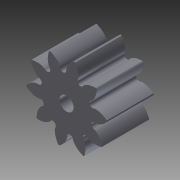
# Autodesk Inventor part: 276-2181-004 Rev1
Saved by Autodesk Inventor 2013 (Build 170138000, 138)
## iProperties
Category: Motors
Company: Autodesk Inc.
Created: 2012-01-24
Part Number: 276-2181-004 Rev1
Material: Steel
Document SubType Name: Modeling
Designer: Autodesk Inc.
Density: 7.85 g/cm^3
Catalog Web Link: http://www.vexrobotics.com/276-2181.html
Vendor: VEX
Mass: 0.321197 g
Surface Area: 1.10628 cm^2
Volume: 0.0409168 cm^3
Author: Autodesk Inc.
Autodesk Inventor part; units mm, degrees
(part 1 of 2)
ref_plane "YZ Plane" through (0, 0, 0) normal (1, 0, 0) x (0, 1, 0)
ref_plane "XZ Plane" through (0, 0, 0) normal (0, 1, 0) x (-1, 0, 0)
ref_plane "XY Plane" through (0, 0, 0) normal (0, 0, 1) x (1, 0, 0)
sketch "Sketch1" plane through (0, 0, 0) normal (0, 0, 1) x (1, 0, 0)
  spline S0 degree 3 poles (1.9335, 1.7383) (1.9334, 1.7374) (1.9328, 1.7292) (1.9315, 1.7139) (1.9295, 1.6925) (1.9272, 1.6714) (1.9247, 1.6506) (1.9219, 1.6301) (1.919, 1.6099) (1.9159, 1.59) (1.9125, 1.5704) (1.909, 1.5512) (1.9053, 1.5323) (1.9014, 1.5137) (1.8974, 1.4954) (1.8932, 1.4775) (1.8888, 1.4598) (1.8843, 1.4426) (1.8797, 1.4256) (1.8749, 1.4089) (1.87, 1.3926) (1.865, 1.3767) (1.8599, 1.361) (1.8547, 1.3457) (1.8494, 1.3307) (1.844, 1.316) (1.8385, 1.3017) (1.833, 1.2877) (1.8274, 1.274) (1.8217, 1.2607) (1.816, 1.2477) (1.8103, 1.235) (1.8045, 1.2226) (1.7987, 1.2106) (1.7928, 1.1989) (1.787, 1.1875) (1.7811, 1.1764) (1.7753, 1.1657) (1.7694, 1.1553) (1.7636, 1.1452) (1.7577, 1.1354) (1.7519, 1.1259) (1.7462, 1.1167) (1.7405, 1.1078) (1.7348, 1.0993) (1.7292, 1.091) (1.7236, 1.083) (1.7181, 1.0754) (1.7127, 1.068) (1.7074, 1.0609) (1.7021, 1.0541) (1.697, 1.0476) (1.6919, 1.0414) (1.687, 1.0355) (1.6821, 1.0298) (1.6774, 1.0244) (1.6728, 1.0193) (1.6683, 1.0144) (1.664, 1.0098) (1.6598, 1.0054) (1.6557, 1.0013) (1.6518, 0.9975) (1.648, 0.9939) (1.6444, 0.9905) (1.641, 0.9874) (1.6378, 0.9845) (1.6347, 0.9818) (1.6318, 0.9793) (1.6291, 0.9771) (1.6266, 0.975) (1.6242, 0.9732) (1.6221, 0.9716) (1.6202, 0.9702) (1.6185, 0.9689) (1.617, 0.9678) (1.6107, 0.9635) (1.5995, 0.9583) (1.585, 0.9495) (1.5719, 0.9412) (1.5594, 0.9325) (1.5474, 0.9234) (1.5359, 0.9137) (1.5249, 0.9036) (1.5144, 0.8928) (1.5044, 0.8812) (1.495, 0.8687) (1.4861, 0.8551) (1.478, 0.8401) (1.4709, 0.8236) (1.4651, 0.8052) (1.461, 0.7849) (1.4595, 0.7627) (1.4612, 0.739) (1.4666, 0.716) (1.4733, 0.6979) (1.4797, 0.6848) (1.4855, 0.6714) (1.495, 0.6545) (1.5091, 0.6356) (1.5261, 0.619) (1.544, 0.6057) (1.562, 0.5956) (1.5798, 0.5882) (1.597, 0.583) (1.6137, 0.5795) (1.6298, 0.5774) (1.6454, 0.5765) (1.6607, 0.5766) (1.6757, 0.5776) (1.6906, 0.5794) (1.7054, 0.5819) (1.7201, 0.5852) (1.7349, 0.5891) (1.7496, 0.5937) (1.7657, 0.5991) (1.7769, 0.6043) (1.7844, 0.6062) (1.7861, 0.6067) (1.7882, 0.6072) (1.7905, 0.6077) (1.7931, 0.6083) (1.796, 0.6089) (1.7992, 0.6095) (1.8027, 0.6101) (1.8064, 0.6107) (1.8105, 0.6113) (1.8148, 0.6119) (1.8194, 0.6125) (1.8243, 0.613) (1.8295, 0.6136) (1.8349, 0.614) (1.8407, 0.6145) (1.8467, 0.6149) (1.853, 0.6152) (1.8596, 0.6155) (1.8665, 0.6157) (1.8737, 0.6158) (1.8812, 0.6158) (1.8889, 0.6157) (1.8969, 0.6156) (1.9052, 0.6153) (1.9138, 0.6149) (1.9227, 0.6144) (1.9318, 0.6137) (1.9412, 0.613) (1.9508, 0.612) (1.9608, 0.611) (1.971, 0.6098) (1.9814, 0.6084) (1.9922, 0.6068) (2.0031, 0.6051) (2.0144, 0.6032) (2.0259, 0.6011) (2.0376, 0.5988) (2.0496, 0.5963) (2.0618, 0.5936) (2.0743, 0.5907) (2.087, 0.5876) (2.0999, 0.5842) (2.1131, 0.5807) (2.1265, 0.5768) (2.1401, 0.5728) (2.1539, 0.5684) (2.168, 0.5639) (2.1823, 0.559) (2.1967, 0.5539) (2.2114, 0.5485) (2.2262, 0.5429) (2.2413, 0.5369) (2.2565, 0.5307) (2.2719, 0.5242) (2.2875, 0.5174) (2.3033, 0.5102) (2.3192, 0.5028) (2.3353, 0.495) (2.3516, 0.4869) (2.368, 0.4785) (2.3845, 0.4698) (2.4012, 0.4607) (2.418, 0.4513) (2.435, 0.4415) (2.4521, 0.4314) (2.4692, 0.4209) (2.4865, 0.4101) (2.5039, 0.3989) (2.5214, 0.3873) (2.539, 0.3754) (2.5574, 0.3626) (2.5699, 0.3536) (2.5765, 0.3488) knots 0.016719 0.016719 0.016719 0.016719 0.017808 0.026543 0.035166 0.043676 0.052073 0.060357 0.068528 0.076587 0.084533 0.092367 0.100087 0.107695 0.115191 0.122573 0.129843 0.137 0.144045 0.150977 0.157796 0.164502 0.171095 0.177576 0.183945 0.1902 0.196343 0.202373 0.20829 0.214095 0.219787 0.225366 0.230832 0.236186 0.241427 0.246556 0.251571 0.256474 0.261264 0.265942 0.270507 0.274959 0.279298 0.283525 0.287639 0.29164 0.295528 0.299304 0.302967 0.306518 0.309956 0.31328 0.316493 0.319592 0.322579 0.325453 0.328215 0.330863 0.333399 0.335823 0.338133 0.340331 0.342416 0.344389 0.346248 0.347996 0.34963 0.351151 0.35256 0.353856 0.35504 0.356111 0.357069 0.357914 0.358647 0.359267 0.367127 0.373439 0.379636 0.385738 0.391769 0.397757 0.403738 0.409752 0.415852 0.422098 0.428563 0.435333 0.442503 0.450171 0.458425 0.467319 0.476841 0.486882 0.495598 0.5 0.504402 0.513118 0.523159 0.532681 0.541575 0.549829 0.557497 0.564667 0.571437 0.577902 0.584148 0.590248 0.596262 0.602243 0.608231 0.614262 0.620364 0.626561 0.632873 0.640733 0.641353 0.642086 0.642931 0.643889 0.64496 0.646144 0.64744 0.648849 0.65037 0.652004 0.653752 0.655611 0.657584 0.659669 0.661867 0.664177 0.666601 0.669137 0.671785 0.674547 0.677421 0.680408 0.683507 0.68672 0.690044 0.693482 0.697033 0.700696 0.704472 0.70836 0.712361 0.716475 0.720702 0.725041 0.729493 0.734058 0.738736 0.743526 0.748429 0.753444 0.758573 0.763814 0.769168 0.774634 0.780213 0.785905 0.79171 0.797627 0.803657 0.8098 0.816055 0.822424 0.828905 0.835498 0.842204 0.849023 0.855955 0.863 0.870157 0.877427 0.884809 0.892305 0.899913 0.907633 0.915467 0.923413 0.931472 0.939643 0.947927 0.956324 0.964834 0.973457 0.983281 0.983281 0.983281 0.983281
  arc A0 (1.9335, 1.7383) -> (1.8794, 1.7966) centre (0, 0) ccw
  spline S1 degree 3 poles (0.5425, 2.5428) (0.543, 2.542) (0.5472, 2.535) (0.5552, 2.5219) (0.5661, 2.5034) (0.5767, 2.4849) (0.5869, 2.4666) (0.5968, 2.4484) (0.6063, 2.4304) (0.6154, 2.4125) (0.6242, 2.3947) (0.6327, 2.377) (0.6408, 2.3596) (0.6486, 2.3422) (0.656, 2.3251) (0.6632, 2.3081) (0.67, 2.2913) (0.6765, 2.2746) (0.6828, 2.2582) (0.6887, 2.2419) (0.6943, 2.2259) (0.6997, 2.21) (0.7047, 2.1943) (0.7095, 2.1789) (0.714, 2.1636) (0.7183, 2.1486) (0.7223, 2.1338) (0.726, 2.1192) (0.7295, 2.1048) (0.7328, 2.0907) (0.7358, 2.0768) (0.7386, 2.0632) (0.7412, 2.0498) (0.7436, 2.0366) (0.7457, 2.0237) (0.7477, 2.0111) (0.7495, 1.9987) (0.751, 1.9865) (0.7524, 1.9747) (0.7536, 1.963) (0.7547, 1.9517) (0.7556, 1.9406) (0.7563, 1.9298) (0.7569, 1.9193) (0.7574, 1.909) (0.7577, 1.899) (0.7579, 1.8893) (0.7579, 1.8799) (0.7579, 1.8707) (0.7577, 1.8619) (0.7575, 1.8533) (0.7571, 1.845) (0.7567, 1.837) (0.7561, 1.8293) (0.7556, 1.8218) (0.7549, 1.8147) (0.7542, 1.8078) (0.7534, 1.8013) (0.7526, 1.795) (0.7518, 1.789) (0.7509, 1.7833) (0.75, 1.7779) (0.7491, 1.7728) (0.7482, 1.7679) (0.7472, 1.7634) (0.7463, 1.7591) (0.7454, 1.7551) (0.7445, 1.7514) (0.7436, 1.748) (0.7428, 1.7449) (0.742, 1.7421) (0.7412, 1.7395) (0.7405, 1.7372) (0.7399, 1.7352) (0.7393, 1.7335) (0.7368, 1.7262) (0.7307, 1.7154) (0.7242, 1.6998) (0.7184, 1.6854) (0.7134, 1.671) (0.7091, 1.6565) (0.7055, 1.642) (0.7026, 1.6273) (0.7004, 1.6124) (0.6992, 1.5972) (0.6989, 1.5815) (0.6997, 1.5653) (0.7019, 1.5484) (0.7059, 1.5309) (0.7119, 1.5126) (0.7206, 1.4938) (0.7325, 1.4749) (0.7478, 1.4567) (0.7656, 1.4413) (0.7817, 1.4306) (0.7946, 1.4237) (0.8072, 1.4164) (0.8247, 1.4083) (0.8473, 1.4012) (0.8708, 1.3977) (0.8931, 1.3976) (0.9136, 1.4) (0.9323, 1.4045) (0.9494, 1.4103) (0.9649, 1.4173) (0.9791, 1.4251) (0.9923, 1.4335) (1.0046, 1.4426) (1.0162, 1.4523) (1.0272, 1.4625) (1.0376, 1.4732) (1.0476, 1.4845) (1.0573, 1.4963) (1.0665, 1.5087) (1.0764, 1.5225) (1.0824, 1.5333) (1.0872, 1.5393) (1.0884, 1.5407) (1.0898, 1.5423) (1.0914, 1.5441) (1.0931, 1.5461) (1.0951, 1.5483) (1.0974, 1.5506) (1.0998, 1.5531) (1.1025, 1.5558) (1.1054, 1.5587) (1.1085, 1.5617) (1.1119, 1.5649) (1.1155, 1.5682) (1.1194, 1.5717) (1.1236, 1.5753) (1.128, 1.5791) (1.1326, 1.5829) (1.1375, 1.5869) (1.1427, 1.591) (1.1482, 1.5952) (1.1539, 1.5995) (1.1599, 1.6039) (1.1662, 1.6084) (1.1728, 1.613) (1.1797, 1.6176) (1.1869, 1.6224) (1.1943, 1.6271) (1.2021, 1.632) (1.2101, 1.6369) (1.2185, 1.6418) (1.2272, 1.6468) (1.2361, 1.6518) (1.2454, 1.6568) (1.255, 1.6619) (1.2649, 1.6669) (1.2751, 1.672) (1.2856, 1.6771) (1.2965, 1.6821) (1.3076, 1.6872) (1.3191, 1.6922) (1.3309, 1.6971) (1.343, 1.7021) (1.3555, 1.707) (1.3682, 1.7118) (1.3813, 1.7166) (1.3947, 1.7213) (1.4085, 1.7259) (1.4225, 1.7305) (1.4369, 1.735) (1.4516, 1.7393) (1.4666, 1.7436) (1.482, 1.7478) (1.4976, 1.7518) (1.5136, 1.7557) (1.5299, 1.7595) (1.5466, 1.7631) (1.5635, 1.7666) (1.5808, 1.77) (1.5984, 1.7731) (1.6163, 1.7762) (1.6345, 1.779) (1.653, 1.7816) (1.6718, 1.7841) (1.691, 1.7864) (1.7104, 1.7884) (1.7302, 1.7903) (1.7502, 1.7919) (1.7706, 1.7933) (1.7912, 1.7945) (1.8122, 1.7954) (1.8334, 1.7961) (1.8559, 1.7965) (1.8712, 1.7966) (1.8794, 1.7966) knots 0.016719 0.016719 0.016719 0.016719 0.017808 0.026543 0.035166 0.043676 0.052073 0.060357 0.068528 0.076587 0.084533 0.092367 0.100087 0.107695 0.115191 0.122573 0.129843 0.137 0.144045 0.150977 0.157796 0.164502 0.171095 0.177576 0.183945 0.1902 0.196343 0.202373 0.20829 0.214095 0.219787 0.225366 0.230832 0.236186 0.241427 0.246556 0.251571 0.256474 0.261264 0.265942 0.270507 0.274959 0.279298 0.283525 0.287639 0.29164 0.295528 0.299304 0.302967 0.306518 0.309956 0.31328 0.316493 0.319592 0.322579 0.325453 0.328215 0.330863 0.333399 0.335823 0.338133 0.340331 0.342416 0.344389 0.346248 0.347996 0.34963 0.351151 0.35256 0.353856 0.35504 0.356111 0.357069 0.357914 0.358647 0.359267 0.367127 0.373439 0.379636 0.385738 0.391769 0.397757 0.403738 0.409752 0.415852 0.422098 0.428563 0.435333 0.442503 0.450171 0.458425 0.467319 0.476841 0.486882 0.495598 0.5 0.504402 0.513118 0.523159 0.532681 0.541575 0.549829 0.557497 0.564667 0.571437 0.577902 0.584148 0.590248 0.596262 0.602243 0.608231 0.614262 0.620364 0.626561 0.632873 0.640733 0.641353 0.642086 0.642931 0.643889 0.64496 0.646144 0.64744 0.648849 0.65037 0.652004 0.653752 0.655611 0.657584 0.659669 0.661867 0.664177 0.666601 0.669137 0.671785 0.674547 0.677421 0.680408 0.683507 0.68672 0.690044 0.693482 0.697033 0.700696 0.704472 0.70836 0.712361 0.716475 0.720702 0.725041 0.729493 0.734058 0.738736 0.743526 0.748429 0.753444 0.758573 0.763814 0.769168 0.774634 0.780213 0.785905 0.79171 0.797627 0.803657 0.8098 0.816055 0.822424 0.828905 0.835498 0.842204 0.849023 0.855955 0.863 0.870157 0.877427 0.884809 0.892305 0.899913 0.907633 0.915467 0.923413 0.931472 0.939643 0.947927 0.956324 0.964834 0.973457 0.983281 0.983281 0.983281 0.983281
  arc A1 (0.5425, 2.5428) -> (0.4644, 2.5582) centre (0, 0) ccw
  spline S2 degree 3 poles (-1.0557, 2.376) (-1.0549, 2.3757) (-1.0473, 2.3726) (-1.0332, 2.3666) (-1.0134, 2.358) (-0.994, 2.3493) (-0.975, 2.3405) (-0.9564, 2.3316) (-0.9381, 2.3226) (-0.9201, 2.3134) (-0.9026, 2.3042) (-0.8854, 2.2949) (-0.8685, 2.2856) (-0.852, 2.2761) (-0.8359, 2.2666) (-0.8201, 2.2571) (-0.8047, 2.2475) (-0.7897, 2.2379) (-0.775, 2.2282) (-0.7606, 2.2186) (-0.7466, 2.2089) (-0.733, 2.1992) (-0.7197, 2.1895) (-0.7067, 2.1798) (-0.6941, 2.1701) (-0.6818, 2.1604) (-0.6699, 2.1508) (-0.6583, 2.1412) (-0.647, 2.1317) (-0.6361, 2.1222) (-0.6254, 2.1127) (-0.6152, 2.1033) (-0.6052, 2.094) (-0.5955, 2.0847) (-0.5862, 2.0756) (-0.5772, 2.0665) (-0.5685, 2.0575) (-0.5601, 2.0486) (-0.552, 2.0398) (-0.5441, 2.0311) (-0.5366, 2.0226) (-0.5294, 2.0141) (-0.5224, 2.0058) (-0.5158, 1.9976) (-0.5094, 1.9896) (-0.5033, 1.9817) (-0.4974, 1.9739) (-0.4918, 1.9664) (-0.4865, 1.9589) (-0.4814, 1.9517) (-0.4766, 1.9446) (-0.472, 1.9377) (-0.4676, 1.9309) (-0.4635, 1.9244) (-0.4596, 1.918) (-0.4559, 1.9118) (-0.4525, 1.9059) (-0.4492, 1.9001) (-0.4462, 1.8946) (-0.4433, 1.8892) (-0.4407, 1.8841) (-0.4382, 1.8792) (-0.436, 1.8745) (-0.4339, 1.87) (-0.432, 1.8658) (-0.4302, 1.8618) (-0.4286, 1.8581) (-0.4271, 1.8546) (-0.4258, 1.8513) (-0.4247, 1.8483) (-0.4237, 1.8455) (-0.4228, 1.843) (-0.422, 1.8407) (-0.4213, 1.8387) (-0.4208, 1.837) (-0.4186, 1.8296) (-0.4171, 1.8173) (-0.4133, 1.8008) (-0.4094, 1.7858) (-0.405, 1.7712) (-0.4, 1.757) (-0.3944, 1.7431) (-0.3881, 1.7295) (-0.3811, 1.7162) (-0.3732, 1.7031) (-0.3642, 1.6902) (-0.354, 1.6776) (-0.3423, 1.6653) (-0.3287, 1.6534) (-0.3131, 1.6422) (-0.295, 1.6321) (-0.2744, 1.6238) (-0.2513, 1.6181) (-0.2278, 1.616) (-0.2084, 1.6168) (-0.194, 1.6189) (-0.1795, 1.6203) (-0.1605, 1.6241) (-0.1381, 1.6316) (-0.1171, 1.6426) (-0.099, 1.6556) (-0.0838, 1.6697) (-0.0712, 1.6843) (-0.0609, 1.699) (-0.0524, 1.7138) (-0.0455, 1.7284) (-0.0398, 1.743) (-0.0352, 1.7576) (-0.0315, 1.7722) (-0.0286, 1.7869) (-0.0265, 1.8017) (-0.025, 1.8167) (-0.0241, 1.832) (-0.0239, 1.8475) (-0.0241, 1.8644) (-0.0256, 1.8767) (-0.0252, 1.8844) (-0.0251, 1.8862) (-0.0249, 1.8883) (-0.0247, 1.8907) (-0.0244, 1.8933) (-0.0241, 1.8963) (-0.0236, 1.8995) (-0.0232, 1.903) (-0.0226, 1.9067) (-0.0219, 1.9108) (-0.0211, 1.915) (-0.0203, 1.9196) (-0.0193, 1.9244) (-0.0182, 1.9295) (-0.017, 1.9349) (-0.0156, 1.9405) (-0.0141, 1.9463) (-0.0125, 1.9525) (-0.0107, 1.9588) (-0.0087, 1.9654) (-0.0066, 1.9723) (-0.0043, 1.9794) (-0.0019, 1.9867) (0.0008, 1.9943) (0.0036, 2.0021) (0.0066, 2.0101) (0.0098, 2.0184) (0.0133, 2.0269) (0.0169, 2.0356) (0.0208, 2.0445) (0.0248, 2.0536) (0.0291, 2.0629) (0.0337, 2.0725) (0.0385, 2.0822) (0.0435, 2.0921) (0.0488, 2.1022) (0.0543, 2.1125) (0.0601, 2.1229) (0.0662, 2.1335) (0.0726, 2.1443) (0.0792, 2.1553) (0.0861, 2.1664) (0.0933, 2.1777) (0.1007, 2.1891) (0.1085, 2.2007) (0.1166, 2.2124) (0.125, 2.2242) (0.1337, 2.2361) (0.1427, 2.2482) (0.152, 2.2604) (0.1617, 2.2727) (0.1716, 2.285) (0.1819, 2.2975) (0.1926, 2.3101) (0.2035, 2.3227) (0.2149, 2.3355) (0.2265, 2.3482) (0.2385, 2.3611) (0.2509, 2.374) (0.2636, 2.387) (0.2767, 2.4) (0.2901, 2.413) (0.3039, 2.4261) (0.318, 2.4391) (0.3326, 2.4522) (0.3474, 2.4653) (0.3627, 2.4785) (0.3784, 2.4916) (0.3944, 2.5046) (0.4108, 2.5177) (0.4276, 2.5307) (0.4454, 2.5443) (0.4578, 2.5534) (0.4644, 2.5582) knots 0.016719 0.016719 0.016719 0.016719 0.017808 0.026543 0.035166 0.043676 0.052073 0.060357 0.068528 0.076587 0.084533 0.092367 0.100087 0.107695 0.115191 0.122573 0.129843 0.137 0.144045 0.150977 0.157796 0.164502 0.171095 0.177576 0.183945 0.1902 0.196343 0.202373 0.20829 0.214095 0.219787 0.225366 0.230832 0.236186 0.241427 0.246556 0.251571 0.256474 0.261264 0.265942 0.270507 0.274959 0.279298 0.283525 0.287639 0.29164 0.295528 0.299304 0.302967 0.306518 0.309956 0.31328 0.316493 0.319592 0.322579 0.325453 0.328215 0.330863 0.333399 0.335823 0.338133 0.340331 0.342416 0.344389 0.346248 0.347996 0.34963 0.351151 0.35256 0.353856 0.35504 0.356111 0.357069 0.357914 0.358647 0.359267 0.367127 0.373439 0.379636 0.385738 0.391769 0.397757 0.403738 0.409752 0.415852 0.422098 0.428563 0.435333 0.442503 0.450171 0.458425 0.467319 0.476841 0.486882 0.495598 0.5 0.504402 0.513118 0.523159 0.532681 0.541575 0.549829 0.557497 0.564667 0.571437 0.577902 0.584148 0.590248 0.596262 0.602243 0.608231 0.614262 0.620364 0.626561 0.632873 0.640733 0.641353 0.642086 0.642931 0.643889 0.64496 0.646144 0.64744 0.648849 0.65037 0.652004 0.653752 0.655611 0.657584 0.659669 0.661867 0.664177 0.666601 0.669137 0.671785 0.674547 0.677421 0.680408 0.683507 0.68672 0.690044 0.693482 0.697033 0.700696 0.704472 0.70836 0.712361 0.716475 0.720702 0.725041 0.729493 0.734058 0.738736 0.743526 0.748429 0.753444 0.758573 0.763814 0.769168 0.774634 0.780213 0.785905 0.79171 0.797627 0.803657 0.8098 0.816055 0.822424 0.828905 0.835498 0.842204 0.849023 0.855955 0.863 0.870157 0.877427 0.884809 0.892305 0.899913 0.907633 0.915467 0.923413 0.931472 0.939643 0.947927 0.956324 0.964834 0.973457 0.983281 0.983281 0.983281 0.983281
  arc A2 (-1.0557, 2.376) -> (-1.1279, 2.3426) centre (0, 0) ccw
  spline S3 degree 3 poles (-2.2507, 1.3017) (-2.2498, 1.3019) (-2.2419, 1.3038) (-2.2269, 1.3073) (-2.2059, 1.312) (-2.1851, 1.3164) (-2.1645, 1.3204) (-2.1442, 1.3242) (-2.1241, 1.3276) (-2.1042, 1.3308) (-2.0846, 1.3336) (-2.0652, 1.3362) (-2.0461, 1.3386) (-2.0272, 1.3406) (-2.0085, 1.3424) (-1.9902, 1.344) (-1.9721, 1.3453) (-1.9542, 1.3463) (-1.9367, 1.3472) (-1.9194, 1.3478) (-1.9024, 1.3482) (-1.8856, 1.3483) (-1.8691, 1.3483) (-1.853, 1.3481) (-1.8371, 1.3477) (-1.8215, 1.3471) (-1.8061, 1.3463) (-1.7911, 1.3454) (-1.7764, 1.3443) (-1.762, 1.343) (-1.7478, 1.3416) (-1.734, 1.34) (-1.7204, 1.3383) (-1.7072, 1.3365) (-1.6942, 1.3346) (-1.6816, 1.3326) (-1.6693, 1.3304) (-1.6572, 1.3281) (-1.6455, 1.3258) (-1.6341, 1.3234) (-1.623, 1.3209) (-1.6121, 1.3183) (-1.6016, 1.3156) (-1.5914, 1.313) (-1.5815, 1.3102) (-1.5719, 1.3074) (-1.5627, 1.3046) (-1.5537, 1.3017) (-1.545, 1.2989) (-1.5366, 1.296) (-1.5285, 1.2931) (-1.5207, 1.2902) (-1.5133, 1.2873) (-1.5061, 1.2844) (-1.4992, 1.2816) (-1.4926, 1.2787) (-1.4863, 1.2759) (-1.4803, 1.2732) (-1.4746, 1.2705) (-1.4691, 1.2678) (-1.464, 1.2652) (-1.4591, 1.2627) (-1.4545, 1.2602) (-1.4502, 1.2579) (-1.4462, 1.2556) (-1.4424, 1.2534) (-1.4389, 1.2513) (-1.4356, 1.2493) (-1.4327, 1.2474) (-1.43, 1.2456) (-1.4275, 1.244) (-1.4253, 1.2425) (-1.4233, 1.2411) (-1.4216, 1.2399) (-1.4202, 1.2388) (-1.414, 1.2342) (-1.4056, 1.2251) (-1.3928, 1.214) (-1.3809, 1.2041) (-1.3687, 1.1949) (-1.3563, 1.1863) (-1.3436, 1.1783) (-1.3306, 1.171) (-1.317, 1.1644) (-1.3029, 1.1585) (-1.2881, 1.1534) (-1.2725, 1.1492) (-1.2557, 1.1461) (-1.2378, 1.1444) (-1.2185, 1.1445) (-1.198, 1.147) (-1.1764, 1.1524) (-1.1544, 1.1613) (-1.1341, 1.1735) (-1.119, 1.1855) (-1.1085, 1.1957) (-1.0976, 1.2054) (-1.0845, 1.2195) (-1.0708, 1.2388) (-1.0602, 1.2601) (-1.0532, 1.2812) (-1.0492, 1.3015) (-1.0476, 1.3207) (-1.0479, 1.3387) (-1.0497, 1.3556) (-1.0528, 1.3716) (-1.0567, 1.3867) (-1.0616, 1.4012) (-1.0672, 1.4152) (-1.0735, 1.4288) (-1.0804, 1.4421) (-1.0881, 1.4551) (-1.0963, 1.4679) (-1.1053, 1.4806) (-1.1154, 1.4942) (-1.1238, 1.5032) (-1.128, 1.5097) (-1.1289, 1.5112) (-1.1301, 1.513) (-1.1313, 1.5151) (-1.1326, 1.5174) (-1.1341, 1.52) (-1.1356, 1.5228) (-1.1373, 1.5259) (-1.139, 1.5293) (-1.1408, 1.5329) (-1.1427, 1.5369) (-1.1447, 1.5411) (-1.1468, 1.5456) (-1.1489, 1.5503) (-1.151, 1.5554) (-1.1532, 1.5607) (-1.1554, 1.5663) (-1.1577, 1.5722) (-1.16, 1.5784) (-1.1623, 1.5849) (-1.1646, 1.5917) (-1.167, 1.5988) (-1.1693, 1.6062) (-1.1716, 1.6139) (-1.1739, 1.6218) (-1.1762, 1.6301) (-1.1784, 1.6387) (-1.1806, 1.6476) (-1.1828, 1.6567) (-1.1849, 1.6662) (-1.187, 1.676) (-1.189, 1.6861) (-1.1909, 1.6965) (-1.1927, 1.7071) (-1.1945, 1.7181) (-1.1961, 1.7294) (-1.1977, 1.741) (-1.1992, 1.7528) (-1.2005, 1.765) (-1.2017, 1.7775) (-1.2028, 1.7902) (-1.2037, 1.8033) (-1.2046, 1.8166) (-1.2052, 1.8302) (-1.2057, 1.8442) (-1.2061, 1.8584) (-1.2062, 1.8729) (-1.2062, 1.8876) (-1.206, 1.9027) (-1.2056, 1.918) (-1.2051, 1.9336) (-1.2043, 1.9495) (-1.2033, 1.9657) (-1.202, 1.9821) (-1.2006, 1.9988) (-1.1989, 2.0157) (-1.197, 2.0329) (-1.1949, 2.0504) (-1.1924, 2.0681) (-1.1898, 2.086) (-1.1868, 2.1042) (-1.1836, 2.1227) (-1.1802, 2.1413) (-1.1764, 2.1602) (-1.1723, 2.1794) (-1.168, 2.1987) (-1.1634, 2.2183) (-1.1584, 2.2381) (-1.1531, 2.2581) (-1.1475, 2.2783) (-1.1416, 2.2987) (-1.1351, 2.3202) (-1.1305, 2.3348) (-1.1279, 2.3426) knots 0.016719 0.016719 0.016719 0.016719 0.017808 0.026543 0.035166 0.043676 0.052073 0.060357 0.068528 0.076587 0.084533 0.092367 0.100087 0.107695 0.115191 0.122573 0.129843 0.137 0.144045 0.150977 0.157796 0.164502 0.171095 0.177576 0.183945 0.1902 0.196343 0.202373 0.20829 0.214095 0.219787 0.225366 0.230832 0.236186 0.241427 0.246556 0.251571 0.256474 0.261264 0.265942 0.270507 0.274959 0.279298 0.283525 0.287639 0.29164 0.295528 0.299304 0.302967 0.306518 0.309956 0.31328 0.316493 0.319592 0.322579 0.325453 0.328215 0.330863 0.333399 0.335823 0.338133 0.340331 0.342416 0.344389 0.346248 0.347996 0.34963 0.351151 0.35256 0.353856 0.35504 0.356111 0.357069 0.357914 0.358647 0.359267 0.367127 0.373439 0.379636 0.385738 0.391769 0.397757 0.403738 0.409752 0.415852 0.422098 0.428563 0.435333 0.442503 0.450171 0.458425 0.467319 0.476841 0.486882 0.495598 0.5 0.504402 0.513118 0.523159 0.532681 0.541575 0.549829 0.557497 0.564667 0.571437 0.577902 0.584148 0.590248 0.596262 0.602243 0.608231 0.614262 0.620364 0.626561 0.632873 0.640733 0.641353 0.642086 0.642931 0.643889 0.64496 0.646144 0.64744 0.648849 0.65037 0.652004 0.653752 0.655611 0.657584 0.659669 0.661867 0.664177 0.666601 0.669137 0.671785 0.674547 0.677421 0.680408 0.683507 0.68672 0.690044 0.693482 0.697033 0.700696 0.704472 0.70836 0.712361 0.716475 0.720702 0.725041 0.729493 0.734058 0.738736 0.743526 0.748429 0.753444 0.758573 0.763814 0.769168 0.774634 0.780213 0.785905 0.79171 0.797627 0.803657 0.8098 0.816055 0.822424 0.828905 0.835498 0.842204 0.849023 0.855955 0.863 0.870157 0.877427 0.884809 0.892305 0.899913 0.907633 0.915467 0.923413 0.931472 0.939643 0.947927 0.956324 0.964834 0.973457 0.983281 0.983281 0.983281 0.983281
  arc A3 (-2.2507, 1.3017) -> (-2.2895, 1.2322) centre (0, 0) ccw
  spline S4 degree 3 poles (-2.586, -0.2698) (-2.5854, -0.2691) (-2.5801, -0.2629) (-2.5701, -0.2513) (-2.5558, -0.2352) (-2.5415, -0.2194) (-2.5273, -0.204) (-2.513, -0.1891) (-2.4988, -0.1744) (-2.4845, -0.1602) (-2.4704, -0.1464) (-2.4562, -0.1329) (-2.4421, -0.1197) (-2.428, -0.107) (-2.414, -0.0946) (-2.4001, -0.0825) (-2.3862, -0.0708) (-2.3724, -0.0595) (-2.3586, -0.0485) (-2.345, -0.0378) (-2.3315, -0.0275) (-2.318, -0.0175) (-2.3047, -0.0078) (-2.2915, 0.0015) (-2.2784, 0.0105) (-2.2654, 0.0192) (-2.2525, 0.0276) (-2.2398, 0.0356) (-2.2273, 0.0434) (-2.2148, 0.0509) (-2.2026, 0.058) (-2.1905, 0.0649) (-2.1785, 0.0715) (-2.1667, 0.0778) (-2.1551, 0.0839) (-2.1437, 0.0896) (-2.1325, 0.0951) (-2.1214, 0.1004) (-2.1105, 0.1054) (-2.0999, 0.1101) (-2.0894, 0.1147) (-2.0791, 0.1189) (-2.0691, 0.123) (-2.0592, 0.1268) (-2.0496, 0.1304) (-2.0402, 0.1338) (-2.031, 0.1369) (-2.0221, 0.1399) (-2.0134, 0.1427) (-2.0049, 0.1453) (-1.9967, 0.1477) (-1.9887, 0.1499) (-1.9809, 0.152) (-1.9734, 0.1539) (-1.9662, 0.1556) (-1.9592, 0.1572) (-1.9524, 0.1586) (-1.9459, 0.1599) (-1.9397, 0.1611) (-1.9338, 0.1622) (-1.9281, 0.1631) (-1.9226, 0.1639) (-1.9175, 0.1646) (-1.9126, 0.1652) (-1.908, 0.1658) (-1.9036, 0.1662) (-1.8996, 0.1666) (-1.8958, 0.1668) (-1.8923, 0.1671) (-1.889, 0.1672) (-1.8861, 0.1674) (-1.8834, 0.1674) (-1.881, 0.1675) (-1.8789, 0.1675) (-1.8771, 0.1675) (-1.8694, 0.1673) (-1.8573, 0.1649) (-1.8404, 0.1634) (-1.8249, 0.1624) (-1.8097, 0.1622) (-1.7946, 0.1625) (-1.7796, 0.1635) (-1.7648, 0.1653) (-1.7499, 0.1679) (-1.735, 0.1714) (-1.72, 0.1759) (-1.7049, 0.1818) (-1.6896, 0.1891) (-1.6741, 0.1983) (-1.6586, 0.2097) (-1.6434, 0.2238) (-1.6291, 0.2408) (-1.6165, 0.261) (-1.6073, 0.2828) (-1.6021, 0.3014) (-1.5996, 0.3158) (-1.5965, 0.33) (-1.5942, 0.3492) (-1.5944, 0.3728) (-1.5984, 0.3963) (-1.6051, 0.4175) (-1.6138, 0.4363) (-1.6238, 0.4527) (-1.6347, 0.4671) (-1.6461, 0.4797) (-1.6579, 0.4908) (-1.67, 0.5007) (-1.6825, 0.5096) (-1.6952, 0.5177) (-1.7083, 0.525) (-1.7217, 0.5316) (-1.7355, 0.5376) (-1.7498, 0.5432) (-1.7644, 0.5481) (-1.7806, 0.5532) (-1.7928, 0.5556) (-1.7999, 0.5584) (-1.8016, 0.559) (-1.8036, 0.5598) (-1.8058, 0.5608) (-1.8082, 0.5619) (-1.8109, 0.5631) (-1.8138, 0.5645) (-1.817, 0.566) (-1.8204, 0.5677) (-1.824, 0.5696) (-1.8279, 0.5717) (-1.8319, 0.5739) (-1.8362, 0.5763) (-1.8407, 0.5789) (-1.8454, 0.5818) (-1.8503, 0.5848) (-1.8554, 0.588) (-1.8607, 0.5915) (-1.8663, 0.5951) (-1.8719, 0.599) (-1.8778, 0.6032) (-1.8839, 0.6075) (-1.8901, 0.6121) (-1.8965, 0.617) (-1.903, 0.6221) (-1.9097, 0.6274) (-1.9166, 0.6331) (-1.9236, 0.6389) (-1.9307, 0.6451) (-1.938, 0.6515) (-1.9454, 0.6582) (-1.953, 0.6652) (-1.9606, 0.6725) (-1.9684, 0.68) (-1.9762, 0.6879) (-1.9842, 0.696) (-1.9923, 0.7045) (-2.0004, 0.7132) (-2.0087, 0.7223) (-2.017, 0.7316) (-2.0253, 0.7413) (-2.0338, 0.7513) (-2.0423, 0.7616) (-2.0508, 0.7723) (-2.0594, 0.7833) (-2.068, 0.7946) (-2.0767, 0.8062) (-2.0854, 0.8181) (-2.0941, 0.8304) (-2.1028, 0.8431) (-2.1115, 0.856) (-2.1202, 0.8693) (-2.1288, 0.883) (-2.1375, 0.897) (-2.1461, 0.9113) (-2.1548, 0.926) (-2.1633, 0.9411) (-2.1718, 0.9565) (-2.1803, 0.9722) (-2.1887, 0.9883) (-2.197, 1.0047) (-2.2053, 1.0215) (-2.2134, 1.0387) (-2.2215, 1.0562) (-2.2295, 1.0741) (-2.2373, 1.0923) (-2.2451, 1.1108) (-2.2527, 1.1298) (-2.2602, 1.1491) (-2.2675, 1.1687) (-2.2747, 1.1887) (-2.2821, 1.2099) (-2.2869, 1.2244) (-2.2895, 1.2322) knots 0.016719 0.016719 0.016719 0.016719 0.017808 0.026543 0.035166 0.043676 0.052073 0.060357 0.068528 0.076587 0.084533 0.092367 0.100087 0.107695 0.115191 0.122573 0.129843 0.137 0.144045 0.150977 0.157796 0.164502 0.171095 0.177576 0.183945 0.1902 0.196343 0.202373 0.20829 0.214095 0.219787 0.225366 0.230832 0.236186 0.241427 0.246556 0.251571 0.256474 0.261264 0.265942 0.270507 0.274959 0.279298 0.283525 0.287639 0.29164 0.295528 0.299304 0.302967 0.306518 0.309956 0.31328 0.316493 0.319592 0.322579 0.325453 0.328215 0.330863 0.333399 0.335823 0.338133 0.340331 0.342416 0.344389 0.346248 0.347996 0.34963 0.351151 0.35256 0.353856 0.35504 0.356111 0.357069 0.357914 0.358647 0.359267 0.367127 0.373439 0.379636 0.385738 0.391769 0.397757 0.403738 0.409752 0.415852 0.422098 0.428563 0.435333 0.442503 0.450171 0.458425 0.467319 0.476841 0.486882 0.495598 0.5 0.504402 0.513118 0.523159 0.532681 0.541575 0.549829 0.557497 0.564667 0.571437 0.577902 0.584148 0.590248 0.596262 0.602243 0.608231 0.614262 0.620364 0.626561 0.632873 0.640733 0.641353 0.642086 0.642931 0.643889 0.64496 0.646144 0.64744 0.648849 0.65037 0.652004 0.653752 0.655611 0.657584 0.659669 0.661867 0.664177 0.666601 0.669137 0.671785 0.674547 0.677421 0.680408 0.683507 0.68672 0.690044 0.693482 0.697033 0.700696 0.704472 0.70836 0.712361 0.716475 0.720702 0.725041 0.729493 0.734058 0.738736 0.743526 0.748429 0.753444 0.758573 0.763814 0.769168 0.774634 0.780213 0.785905 0.79171 0.797627 0.803657 0.8098 0.816055 0.822424 0.828905 0.835498 0.842204 0.849023 0.855955 0.863 0.870157 0.877427 0.884809 0.892305 0.899913 0.907633 0.915467 0.923413 0.931472 0.939643 0.947927 0.956324 0.964834 0.973457 0.983281 0.983281 0.983281 0.983281
  arc A4 (-2.586, -0.2698) -> (-2.5765, -0.3488) centre (0, 0) ccw
  spline S5 degree 3 poles (-1.9335, -1.7383) (-1.9334, -1.7374) (-1.9328, -1.7292) (-1.9315, -1.7139) (-1.9295, -1.6925) (-1.9272, -1.6714) (-1.9247, -1.6506) (-1.9219, -1.6301) (-1.919, -1.6099) (-1.9159, -1.59) (-1.9125, -1.5704) (-1.909, -1.5512) (-1.9053, -1.5323) (-1.9014, -1.5137) (-1.8974, -1.4954) (-1.8932, -1.4775) (-1.8888, -1.4598) (-1.8843, -1.4426) (-1.8797, -1.4256) (-1.8749, -1.4089) (-1.87, -1.3926) (-1.865, -1.3767) (-1.8599, -1.361) (-1.8547, -1.3457) (-1.8494, -1.3307) (-1.844, -1.316) (-1.8385, -1.3017) (-1.833, -1.2877) (-1.8274, -1.274) (-1.8217, -1.2607) (-1.816, -1.2477) (-1.8103, -1.235) (-1.8045, -1.2226) (-1.7987, -1.2106) (-1.7928, -1.1989) (-1.787, -1.1875) (-1.7811, -1.1764) (-1.7753, -1.1657) (-1.7694, -1.1553) (-1.7636, -1.1452) (-1.7577, -1.1354) (-1.7519, -1.1259) (-1.7462, -1.1167) (-1.7405, -1.1078) (-1.7348, -1.0993) (-1.7292, -1.091) (-1.7236, -1.083) (-1.7181, -1.0754) (-1.7127, -1.068) (-1.7074, -1.0609) (-1.7021, -1.0541) (-1.697, -1.0476) (-1.6919, -1.0414) (-1.687, -1.0355) (-1.6821, -1.0298) (-1.6774, -1.0244) (-1.6728, -1.0193) (-1.6683, -1.0144) (-1.664, -1.0098) (-1.6598, -1.0054) (-1.6557, -1.0013) (-1.6518, -0.9975) (-1.648, -0.9939) (-1.6444, -0.9905) (-1.641, -0.9874) (-1.6378, -0.9845) (-1.6347, -0.9818) (-1.6318, -0.9793) (-1.6291, -0.9771) (-1.6266, -0.975) (-1.6242, -0.9732) (-1.6221, -0.9716) (-1.6202, -0.9702) (-1.6185, -0.9689) (-1.617, -0.9678) (-1.6107, -0.9635) (-1.5995, -0.9583) (-1.585, -0.9495) (-1.5719, -0.9412) (-1.5594, -0.9325) (-1.5474, -0.9234) (-1.5359, -0.9137) (-1.5249, -0.9036) (-1.5144, -0.8928) (-1.5044, -0.8812) (-1.495, -0.8687) (-1.4861, -0.8551) (-1.478, -0.8401) (-1.4709, -0.8236) (-1.4651, -0.8052) (-1.461, -0.7849) (-1.4595, -0.7627) (-1.4612, -0.739) (-1.4666, -0.716) (-1.4733, -0.6979) (-1.4797, -0.6848) (-1.4855, -0.6714) (-1.495, -0.6546) (-1.5091, -0.6356) (-1.5261, -0.619) (-1.544, -0.6057) (-1.562, -0.5956) (-1.5798, -0.5882) (-1.597, -0.583) (-1.6137, -0.5795) (-1.6298, -0.5774) (-1.6454, -0.5765) (-1.6607, -0.5766) (-1.6757, -0.5776) (-1.6906, -0.5794) (-1.7054, -0.5819) (-1.7201, -0.5852) (-1.7349, -0.5891) (-1.7496, -0.5937) (-1.7657, -0.5991) (-1.7769, -0.6043) (-1.7844, -0.6062) (-1.7861, -0.6067) (-1.7882, -0.6072) (-1.7905, -0.6077) (-1.7931, -0.6083) (-1.796, -0.6089) (-1.7992, -0.6095) (-1.8027, -0.6101) (-1.8064, -0.6107) (-1.8105, -0.6113) (-1.8148, -0.6119) (-1.8194, -0.6125) (-1.8243, -0.613) (-1.8295, -0.6136) (-1.8349, -0.614) (-1.8407, -0.6145) (-1.8467, -0.6149) (-1.853, -0.6152) (-1.8596, -0.6155) (-1.8665, -0.6157) (-1.8737, -0.6158) (-1.8812, -0.6158) (-1.8889, -0.6157) (-1.8969, -0.6156) (-1.9052, -0.6153) (-1.9138, -0.6149) (-1.9226, -0.6144) (-1.9318, -0.6137) (-1.9412, -0.613) (-1.9508, -0.612) (-1.9608, -0.611) (-1.971, -0.6098) (-1.9814, -0.6084) (-1.9922, -0.6068) (-2.0031, -0.6051) (-2.0144, -0.6032) (-2.0259, -0.6011) (-2.0376, -0.5988) (-2.0496, -0.5963) (-2.0618, -0.5936) (-2.0743, -0.5907) (-2.087, -0.5876) (-2.0999, -0.5842) (-2.1131, -0.5807) (-2.1265, -0.5768) (-2.1401, -0.5728) (-2.1539, -0.5684) (-2.168, -0.5639) (-2.1822, -0.559) (-2.1967, -0.5539) (-2.2114, -0.5485) (-2.2262, -0.5429) (-2.2413, -0.5369) (-2.2565, -0.5307) (-2.2719, -0.5242) (-2.2875, -0.5174) (-2.3033, -0.5102) (-2.3192, -0.5028) (-2.3353, -0.495) (-2.3516, -0.4869) (-2.368, -0.4785) (-2.3845, -0.4698) (-2.4012, -0.4607) (-2.418, -0.4513) (-2.435, -0.4415) (-2.452, -0.4314) (-2.4692, -0.4209) (-2.4865, -0.4101) (-2.5039, -0.3989) (-2.5214, -0.3873) (-2.539, -0.3754) (-2.5574, -0.3626) (-2.5699, -0.3536) (-2.5765, -0.3488) knots 0.016719 0.016719 0.016719 0.016719 0.017808 0.026543 0.035166 0.043676 0.052073 0.060357 0.068528 0.076587 0.084533 0.092367 0.100087 0.107695 0.115191 0.122573 0.129843 0.137 0.144045 0.150977 0.157796 0.164502 0.171095 0.177576 0.183945 0.1902 0.196343 0.202373 0.20829 0.214095 0.219787 0.225366 0.230832 0.236186 0.241427 0.246556 0.251571 0.256474 0.261264 0.265942 0.270507 0.274959 0.279298 0.283525 0.287639 0.29164 0.295528 0.299304 0.302967 0.306518 0.309956 0.31328 0.316493 0.319592 0.322579 0.325453 0.328215 0.330863 0.333399 0.335823 0.338133 0.340331 0.342416 0.344389 0.346248 0.347996 0.34963 0.351151 0.35256 0.353856 0.35504 0.356111 0.357069 0.357914 0.358647 0.359267 0.367127 0.373439 0.379636 0.385738 0.391769 0.397757 0.403738 0.409752 0.415852 0.422098 0.428563 0.435333 0.442503 0.450171 0.458425 0.467319 0.476841 0.486882 0.495598 0.5 0.504402 0.513118 0.523159 0.532681 0.541575 0.549829 0.557497 0.564667 0.571437 0.577902 0.584148 0.590248 0.596262 0.602243 0.608231 0.614262 0.620364 0.626561 0.632873 0.640733 0.641353 0.642086 0.642931 0.643889 0.64496 0.646144 0.64744 0.648849 0.65037 0.652004 0.653752 0.655611 0.657584 0.659669 0.661867 0.664177 0.666601 0.669137 0.671785 0.674547 0.677421 0.680408 0.683507 0.68672 0.690044 0.693482 0.697033 0.700696 0.704472 0.70836 0.712361 0.716475 0.720702 0.725041 0.729493 0.734058 0.738736 0.743526 0.748429 0.753444 0.758573 0.763814 0.769168 0.774634 0.780213 0.785905 0.79171 0.797627 0.803657 0.8098 0.816055 0.822424 0.828905 0.835498 0.842204 0.849023 0.855955 0.863 0.870157 0.877427 0.884809 0.892305 0.899913 0.907633 0.915467 0.923413 0.931472 0.939643 0.947927 0.956324 0.964834 0.973457 0.983281 0.983281 0.983281 0.983281
  arc A5 (-1.9335, -1.7383) -> (-1.8794, -1.7966) centre (0, 0) ccw
  spline S6 degree 3 poles (-0.5425, -2.5428) (-0.543, -2.542) (-0.5472, -2.535) (-0.5552, -2.5219) (-0.5661, -2.5034) (-0.5767, -2.4849) (-0.5869, -2.4666) (-0.5968, -2.4484) (-0.6063, -2.4304) (-0.6154, -2.4125) (-0.6242, -2.3947) (-0.6327, -2.377) (-0.6408, -2.3596) (-0.6486, -2.3422) (-0.656, -2.3251) (-0.6632, -2.3081) (-0.67, -2.2913) (-0.6765, -2.2746) (-0.6828, -2.2582) (-0.6887, -2.2419) (-0.6943, -2.2259) (-0.6997, -2.21) (-0.7047, -2.1943) (-0.7095, -2.1789) (-0.714, -2.1636) (-0.7183, -2.1486) (-0.7223, -2.1338) (-0.726, -2.1192) (-0.7295, -2.1048) (-0.7328, -2.0907) (-0.7358, -2.0768) (-0.7386, -2.0632) (-0.7412, -2.0498) (-0.7436, -2.0366) (-0.7457, -2.0237) (-0.7477, -2.0111) (-0.7495, -1.9987) (-0.751, -1.9865) (-0.7524, -1.9747) (-0.7536, -1.963) (-0.7547, -1.9517) (-0.7556, -1.9406) (-0.7563, -1.9298) (-0.7569, -1.9193) (-0.7574, -1.909) (-0.7577, -1.899) (-0.7579, -1.8893) (-0.7579, -1.8799) (-0.7579, -1.8707) (-0.7577, -1.8619) (-0.7575, -1.8533) (-0.7571, -1.845) (-0.7567, -1.837) (-0.7561, -1.8293) (-0.7556, -1.8218) (-0.7549, -1.8147) (-0.7542, -1.8078) (-0.7534, -1.8013) (-0.7526, -1.795) (-0.7518, -1.789) (-0.7509, -1.7833) (-0.75, -1.7779) (-0.7491, -1.7728) (-0.7482, -1.7679) (-0.7472, -1.7634) (-0.7463, -1.7591) (-0.7454, -1.7551) (-0.7445, -1.7514) (-0.7436, -1.748) (-0.7428, -1.7449) (-0.742, -1.7421) (-0.7412, -1.7395) (-0.7405, -1.7372) (-0.7399, -1.7352) (-0.7393, -1.7335) (-0.7368, -1.7262) (-0.7307, -1.7154) (-0.7242, -1.6998) (-0.7184, -1.6854) (-0.7134, -1.671) (-0.7091, -1.6565) (-0.7055, -1.642) (-0.7026, -1.6273) (-0.7004, -1.6124) (-0.6992, -1.5972) (-0.6989, -1.5815) (-0.6997, -1.5653) (-0.7019, -1.5484) (-0.7059, -1.5309) (-0.7119, -1.5126) (-0.7206, -1.4938) (-0.7325, -1.4749) (-0.7478, -1.4567) (-0.7656, -1.4413) (-0.7817, -1.4306) (-0.7946, -1.4237) (-0.8072, -1.4164) (-0.8247, -1.4083) (-0.8473, -1.4012) (-0.8708, -1.3977) (-0.8931, -1.3976) (-0.9136, -1.4) (-0.9323, -1.4045) (-0.9494, -1.4103) (-0.9649, -1.4173) (-0.9791, -1.4251) (-0.9923, -1.4335) (-1.0046, -1.4426) (-1.0162, -1.4523) (-1.0272, -1.4625) (-1.0376, -1.4732) (-1.0476, -1.4845) (-1.0573, -1.4963) (-1.0665, -1.5087) (-1.0764, -1.5225) (-1.0824, -1.5333) (-1.0872, -1.5393) (-1.0884, -1.5407) (-1.0898, -1.5423) (-1.0914, -1.5441) (-1.0931, -1.5461) (-1.0951, -1.5483) (-1.0974, -1.5506) (-1.0998, -1.5531) (-1.1025, -1.5558) (-1.1054, -1.5587) (-1.1085, -1.5617) (-1.1119, -1.5649) (-1.1155, -1.5682) (-1.1194, -1.5717) (-1.1236, -1.5753) (-1.128, -1.5791) (-1.1326, -1.5829) (-1.1375, -1.5869) (-1.1427, -1.591) (-1.1482, -1.5952) (-1.1539, -1.5995) (-1.1599, -1.6039) (-1.1662, -1.6084) (-1.1728, -1.613) (-1.1797, -1.6176) (-1.1869, -1.6224) (-1.1943, -1.6271) (-1.2021, -1.632) (-1.2101, -1.6369) (-1.2185, -1.6418) (-1.2272, -1.6468) (-1.2361, -1.6518) (-1.2454, -1.6568) (-1.255, -1.6619) (-1.2649, -1.6669) (-1.2751, -1.672) (-1.2856, -1.6771) (-1.2965, -1.6821) (-1.3076, -1.6872) (-1.3191, -1.6922) (-1.3309, -1.6971) (-1.343, -1.7021) (-1.3555, -1.707) (-1.3682, -1.7118) (-1.3813, -1.7166) (-1.3947, -1.7213) (-1.4085, -1.7259) (-1.4225, -1.7305) (-1.4369, -1.735) (-1.4516, -1.7393) (-1.4666, -1.7436) (-1.482, -1.7478) (-1.4976, -1.7518) (-1.5136, -1.7557) (-1.5299, -1.7595) (-1.5466, -1.7631) (-1.5635, -1.7666) (-1.5808, -1.77) (-1.5984, -1.7731) (-1.6163, -1.7762) (-1.6345, -1.779) (-1.653, -1.7816) (-1.6718, -1.7841) (-1.691, -1.7864) (-1.7104, -1.7884) (-1.7302, -1.7903) (-1.7502, -1.7919) (-1.7706, -1.7933) (-1.7912, -1.7945) (-1.8122, -1.7954) (-1.8334, -1.7961) (-1.8559, -1.7965) (-1.8712, -1.7966) (-1.8794, -1.7966) knots 0.016719 0.016719 0.016719 0.016719 0.017808 0.026543 0.035166 0.043676 0.052073 0.060357 0.068528 0.076587 0.084533 0.092367 0.100087 0.107695 0.115191 0.122573 0.129843 0.137 0.144045 0.150977 0.157796 0.164502 0.171095 0.177576 0.183945 0.1902 0.196343 0.202373 0.20829 0.214095 0.219787 0.225366 0.230832 0.236186 0.241427 0.246556 0.251571 0.256474 0.261264 0.265942 0.270507 0.274959 0.279298 0.283525 0.287639 0.29164 0.295528 0.299304 0.302967 0.306518 0.309956 0.31328 0.316493 0.319592 0.322579 0.325453 0.328215 0.330863 0.333399 0.335823 0.338133 0.340331 0.342416 0.344389 0.346248 0.347996 0.34963 0.351151 0.35256 0.353856 0.35504 0.356111 0.357069 0.357914 0.358647 0.359267 0.367127 0.373439 0.379636 0.385738 0.391769 0.397757 0.403738 0.409752 0.415852 0.422098 0.428563 0.435333 0.442503 0.450171 0.458425 0.467319 0.476841 0.486882 0.495598 0.5 0.504402 0.513118 0.523159 0.532681 0.541575 0.549829 0.557497 0.564667 0.571437 0.577902 0.584148 0.590248 0.596262 0.602243 0.608231 0.614262 0.620364 0.626561 0.632873 0.640733 0.641353 0.642086 0.642931 0.643889 0.64496 0.646144 0.64744 0.648849 0.65037 0.652004 0.653752 0.655611 0.657584 0.659669 0.661867 0.664177 0.666601 0.669137 0.671785 0.674547 0.677421 0.680408 0.683507 0.68672 0.690044 0.693482 0.697033 0.700696 0.704472 0.70836 0.712361 0.716475 0.720702 0.725041 0.729493 0.734058 0.738736 0.743526 0.748429 0.753444 0.758573 0.763814 0.769168 0.774634 0.780213 0.785905 0.79171 0.797627 0.803657 0.8098 0.816055 0.822424 0.828905 0.835498 0.842204 0.849023 0.855955 0.863 0.870157 0.877427 0.884809 0.892305 0.899913 0.907633 0.915467 0.923413 0.931472 0.939643 0.947927 0.956324 0.964834 0.973457 0.983281 0.983281 0.983281 0.983281
  arc A6 (-0.5425, -2.5428) -> (-0.4644, -2.5582) centre (0, 0) ccw
  spline S7 degree 3 poles (1.0557, -2.376) (1.0549, -2.3757) (1.0473, -2.3726) (1.0332, -2.3666) (1.0134, -2.358) (0.994, -2.3493) (0.975, -2.3405) (0.9564, -2.3316) (0.9381, -2.3226) (0.9201, -2.3134) (0.9026, -2.3042) (0.8854, -2.2949) (0.8685, -2.2856) (0.852, -2.2761) (0.8359, -2.2666) (0.8201, -2.2571) (0.8047, -2.2475) (0.7897, -2.2379) (0.775, -2.2282) (0.7606, -2.2186) (0.7466, -2.2089) (0.733, -2.1992) (0.7197, -2.1895) (0.7067, -2.1798) (0.6941, -2.1701) (0.6818, -2.1604) (0.6699, -2.1508) (0.6583, -2.1412) (0.647, -2.1317) (0.6361, -2.1222) (0.6254, -2.1127) (0.6152, -2.1033) (0.6052, -2.094) (0.5955, -2.0847) (0.5862, -2.0756) (0.5772, -2.0665) (0.5685, -2.0575) (0.5601, -2.0486) (0.552, -2.0398) (0.5441, -2.0311) (0.5366, -2.0226) (0.5294, -2.0141) (0.5224, -2.0058) (0.5158, -1.9976) (0.5094, -1.9896) (0.5033, -1.9817) (0.4974, -1.9739) (0.4918, -1.9664) (0.4865, -1.9589) (0.4814, -1.9517) (0.4766, -1.9446) (0.472, -1.9377) (0.4676, -1.9309) (0.4635, -1.9244) (0.4596, -1.918) (0.4559, -1.9118) (0.4525, -1.9059) (0.4492, -1.9001) (0.4462, -1.8946) (0.4433, -1.8892) (0.4407, -1.8841) (0.4382, -1.8792) (0.436, -1.8745) (0.4339, -1.87) (0.432, -1.8658) (0.4302, -1.8618) (0.4286, -1.8581) (0.4271, -1.8546) (0.4258, -1.8513) (0.4247, -1.8483) (0.4237, -1.8455) (0.4228, -1.843) (0.422, -1.8407) (0.4213, -1.8387) (0.4208, -1.837) (0.4186, -1.8296) (0.4171, -1.8173) (0.4133, -1.8008) (0.4094, -1.7858) (0.405, -1.7712) (0.4, -1.757) (0.3944, -1.7431) (0.3881, -1.7295) (0.3811, -1.7161) (0.3732, -1.7031) (0.3642, -1.6902) (0.354, -1.6776) (0.3423, -1.6653) (0.3287, -1.6534) (0.3131, -1.6422) (0.295, -1.6321) (0.2744, -1.6238) (0.2513, -1.6181) (0.2278, -1.616) (0.2084, -1.6168) (0.194, -1.6189) (0.1795, -1.6203) (0.1605, -1.6241) (0.1381, -1.6316) (0.1171, -1.6426) (0.099, -1.6556) (0.0838, -1.6697) (0.0712, -1.6843) (0.0609, -1.699) (0.0524, -1.7138) (0.0455, -1.7284) (0.0398, -1.743) (0.0352, -1.7576) (0.0315, -1.7722) (0.0286, -1.7869) (0.0265, -1.8017) (0.025, -1.8167) (0.0241, -1.832) (0.0239, -1.8475) (0.0241, -1.8644) (0.0256, -1.8767) (0.0252, -1.8844) (0.0251, -1.8862) (0.0249, -1.8883) (0.0247, -1.8907) (0.0244, -1.8933) (0.0241, -1.8963) (0.0236, -1.8995) (0.0232, -1.903) (0.0226, -1.9067) (0.0219, -1.9107) (0.0211, -1.915) (0.0203, -1.9196) (0.0193, -1.9244) (0.0182, -1.9295) (0.017, -1.9349) (0.0156, -1.9405) (0.0141, -1.9463) (0.0125, -1.9525) (0.0107, -1.9588) (0.0087, -1.9654) (0.0066, -1.9723) (0.0043, -1.9794) (0.0019, -1.9867) (-0.0008, -1.9943) (-0.0036, -2.0021) (-0.0066, -2.0101) (-0.0098, -2.0184) (-0.0133, -2.0269) (-0.0169, -2.0356) (-0.0208, -2.0445) (-0.0248, -2.0536) (-0.0291, -2.0629) (-0.0337, -2.0724) (-0.0385, -2.0822) (-0.0435, -2.0921) (-0.0488, -2.1022) (-0.0543, -2.1125) (-0.0601, -2.1229) (-0.0662, -2.1335) (-0.0726, -2.1443) (-0.0792, -2.1553) (-0.0861, -2.1664) (-0.0933, -2.1777) (-0.1007, -2.1891) (-0.1085, -2.2007) (-0.1166, -2.2124) (-0.125, -2.2242) (-0.1337, -2.2361) (-0.1427, -2.2482) (-0.152, -2.2604) (-0.1617, -2.2727) (-0.1716, -2.285) (-0.1819, -2.2975) (-0.1926, -2.3101) (-0.2035, -2.3227) (-0.2149, -2.3355) (-0.2265, -2.3482) (-0.2385, -2.3611) (-0.2509, -2.374) (-0.2636, -2.387) (-0.2767, -2.4) (-0.2901, -2.413) (-0.3039, -2.4261) (-0.318, -2.4391) (-0.3326, -2.4522) (-0.3474, -2.4653) (-0.3627, -2.4784) (-0.3784, -2.4915) (-0.3944, -2.5046) (-0.4108, -2.5177) (-0.4276, -2.5307) (-0.4454, -2.5443) (-0.4578, -2.5534) (-0.4644, -2.5582) knots 0.016719 0.016719 0.016719 0.016719 0.017808 0.026543 0.035166 0.043676 0.052073 0.060357 0.068528 0.076587 0.084533 0.092367 0.100087 0.107695 0.115191 0.122573 0.129843 0.137 0.144045 0.150977 0.157796 0.164502 0.171095 0.177576 0.183945 0.1902 0.196343 0.202373 0.20829 0.214095 0.219787 0.225366 0.230832 0.236186 0.241427 0.246556 0.251571 0.256474 0.261264 0.265942 0.270507 0.274959 0.279298 0.283525 0.287639 0.29164 0.295528 0.299304 0.302967 0.306518 0.309956 0.31328 0.316493 0.319592 0.322579 0.325453 0.328215 0.330863 0.333399 0.335823 0.338133 0.340331 0.342416 0.344389 0.346248 0.347996 0.34963 0.351151 0.35256 0.353856 0.35504 0.356111 0.357069 0.357914 0.358647 0.359267 0.367127 0.373439 0.379636 0.385738 0.391769 0.397757 0.403738 0.409752 0.415852 0.422098 0.428563 0.435333 0.442503 0.450171 0.458425 0.467319 0.476841 0.486882 0.495598 0.5 0.504402 0.513118 0.523159 0.532681 0.541575 0.549829 0.557497 0.564667 0.571437 0.577902 0.584148 0.590248 0.596262 0.602243 0.608231 0.614262 0.620364 0.626561 0.632873 0.640733 0.641353 0.642086 0.642931 0.643889 0.64496 0.646144 0.64744 0.648849 0.65037 0.652004 0.653752 0.655611 0.657584 0.659669 0.661867 0.664177 0.666601 0.669137 0.671785 0.674547 0.677421 0.680408 0.683507 0.68672 0.690044 0.693482 0.697033 0.700696 0.704472 0.70836 0.712361 0.716475 0.720702 0.725041 0.729493 0.734058 0.738736 0.743526 0.748429 0.753444 0.758573 0.763814 0.769168 0.774634 0.780213 0.785905 0.79171 0.797627 0.803657 0.8098 0.816055 0.822424 0.828905 0.835498 0.842204 0.849023 0.855955 0.863 0.870157 0.877427 0.884809 0.892305 0.899913 0.907633 0.915467 0.923413 0.931472 0.939643 0.947927 0.956324 0.964834 0.973457 0.983281 0.983281 0.983281 0.983281
  arc A7 (1.0557, -2.376) -> (1.1279, -2.3426) centre (0, 0) ccw
  spline S8 degree 3 poles (2.2507, -1.3017) (2.2498, -1.3019) (2.2419, -1.3038) (2.2269, -1.3073) (2.2059, -1.312) (2.1851, -1.3164) (2.1645, -1.3204) (2.1442, -1.3242) (2.1241, -1.3276) (2.1042, -1.3308) (2.0846, -1.3336) (2.0652, -1.3362) (2.0461, -1.3386) (2.0272, -1.3406) (2.0085, -1.3424) (1.9902, -1.344) (1.9721, -1.3453) (1.9542, -1.3463) (1.9367, -1.3472) (1.9194, -1.3478) (1.9024, -1.3482) (1.8856, -1.3483) (1.8691, -1.3483) (1.853, -1.3481) (1.8371, -1.3477) (1.8215, -1.3471) (1.8061, -1.3463) (1.7911, -1.3454) (1.7764, -1.3443) (1.762, -1.343) (1.7478, -1.3416) (1.734, -1.34) (1.7204, -1.3383) (1.7072, -1.3365) (1.6942, -1.3346) (1.6816, -1.3326) (1.6693, -1.3304) (1.6572, -1.3281) (1.6455, -1.3258) (1.6341, -1.3234) (1.623, -1.3209) (1.6121, -1.3183) (1.6016, -1.3156) (1.5914, -1.313) (1.5815, -1.3102) (1.5719, -1.3074) (1.5627, -1.3046) (1.5537, -1.3017) (1.545, -1.2989) (1.5366, -1.296) (1.5285, -1.2931) (1.5207, -1.2902) (1.5133, -1.2873) (1.5061, -1.2844) (1.4992, -1.2816) (1.4926, -1.2787) (1.4863, -1.2759) (1.4803, -1.2732) (1.4746, -1.2705) (1.4691, -1.2678) (1.464, -1.2652) (1.4591, -1.2627) (1.4545, -1.2602) (1.4502, -1.2579) (1.4462, -1.2556) (1.4424, -1.2534) (1.4389, -1.2513) (1.4356, -1.2493) (1.4327, -1.2474) (1.43, -1.2456) (1.4275, -1.244) (1.4253, -1.2425) (1.4233, -1.2411) (1.4216, -1.2399) (1.4202, -1.2388) (1.414, -1.2342) (1.4056, -1.2251) (1.3928, -1.214) (1.3809, -1.2041) (1.3687, -1.1949) (1.3563, -1.1863) (1.3436, -1.1783) (1.3306, -1.171) (1.317, -1.1644) (1.3029, -1.1585) (1.2881, -1.1534) (1.2725, -1.1492) (1.2557, -1.1461) (1.2378, -1.1444) (1.2185, -1.1445) (1.198, -1.147) (1.1764, -1.1524) (1.1544, -1.1613) (1.1341, -1.1735) (1.119, -1.1855) (1.1085, -1.1957) (1.0976, -1.2054) (1.0845, -1.2195) (1.0708, -1.2388) (1.0602, -1.2601) (1.0532, -1.2812) (1.0492, -1.3015) (1.0476, -1.3207) (1.0479, -1.3387) (1.0497, -1.3556) (1.0528, -1.3716) (1.0567, -1.3867) (1.0616, -1.4012) (1.0672, -1.4152) (1.0735, -1.4288) (1.0804, -1.4421) (1.0881, -1.4551) (1.0963, -1.4679) (1.1053, -1.4806) (1.1154, -1.4942) (1.1238, -1.5032) (1.128, -1.5097) (1.1289, -1.5112) (1.1301, -1.513) (1.1313, -1.5151) (1.1326, -1.5174) (1.1341, -1.52) (1.1356, -1.5228) (1.1373, -1.5259) (1.139, -1.5293) (1.1408, -1.5329) (1.1427, -1.5369) (1.1447, -1.5411) (1.1468, -1.5456) (1.1489, -1.5503) (1.151, -1.5554) (1.1532, -1.5607) (1.1554, -1.5663) (1.1577, -1.5722) (1.16, -1.5784) (1.1623, -1.5849) (1.1646, -1.5917) (1.167, -1.5988) (1.1693, -1.6062) (1.1716, -1.6139) (1.1739, -1.6218) (1.1762, -1.6301) (1.1784, -1.6387) (1.1806, -1.6476) (1.1828, -1.6567) (1.1849, -1.6662) (1.187, -1.676) (1.189, -1.6861) (1.1909, -1.6965) (1.1927, -1.7071) (1.1945, -1.7181) (1.1961, -1.7294) (1.1977, -1.741) (1.1992, -1.7528) (1.2005, -1.765) (1.2017, -1.7775) (1.2028, -1.7902) (1.2037, -1.8033) (1.2046, -1.8166) (1.2052, -1.8302) (1.2057, -1.8442) (1.2061, -1.8584) (1.2062, -1.8729) (1.2062, -1.8876) (1.206, -1.9027) (1.2056, -1.918) (1.2051, -1.9336) (1.2043, -1.9495) (1.2033, -1.9657) (1.202, -1.9821) (1.2006, -1.9988) (1.1989, -2.0157) (1.197, -2.0329) (1.1949, -2.0504) (1.1924, -2.0681) (1.1898, -2.086) (1.1868, -2.1042) (1.1836, -2.1227) (1.1802, -2.1413) (1.1764, -2.1602) (1.1723, -2.1794) (1.168, -2.1987) (1.1634, -2.2183) (1.1584, -2.2381) (1.1531, -2.2581) (1.1475, -2.2783) (1.1416, -2.2987) (1.1351, -2.3202) (1.1305, -2.3348) (1.1279, -2.3426) knots 0.016719 0.016719 0.016719 0.016719 0.017808 0.026543 0.035166 0.043676 0.052073 0.060357 0.068528 0.076587 0.084533 0.092367 0.100087 0.107695 0.115191 0.122573 0.129843 0.137 0.144045 0.150977 0.157796 0.164502 0.171095 0.177576 0.183945 0.1902 0.196343 0.202373 0.20829 0.214095 0.219787 0.225366 0.230832 0.236186 0.241427 0.246556 0.251571 0.256474 0.261264 0.265942 0.270507 0.274959 0.279298 0.283525 0.287639 0.29164 0.295528 0.299304 0.302967 0.306518 0.309956 0.31328 0.316493 0.319592 0.322579 0.325453 0.328215 0.330863 0.333399 0.335823 0.338133 0.340331 0.342416 0.344389 0.346248 0.347996 0.34963 0.351151 0.35256 0.353856 0.35504 0.356111 0.357069 0.357914 0.358647 0.359267 0.367127 0.373439 0.379636 0.385738 0.391769 0.397757 0.403738 0.409752 0.415852 0.422098 0.428563 0.435333 0.442503 0.450171 0.458425 0.467319 0.476841 0.486882 0.495598 0.5 0.504402 0.513118 0.523159 0.532681 0.541575 0.549829 0.557497 0.564667 0.571437 0.577902 0.584148 0.590248 0.596262 0.602243 0.608231 0.614262 0.620364 0.626561 0.632873 0.640733 0.641353 0.642086 0.642931 0.643889 0.64496 0.646144 0.64744 0.648849 0.65037 0.652004 0.653752 0.655611 0.657584 0.659669 0.661867 0.664177 0.666601 0.669137 0.671785 0.674547 0.677421 0.680408 0.683507 0.68672 0.690044 0.693482 0.697033 0.700696 0.704472 0.70836 0.712361 0.716475 0.720702 0.725041 0.729493 0.734058 0.738736 0.743526 0.748429 0.753444 0.758573 0.763814 0.769168 0.774634 0.780213 0.785905 0.79171 0.797627 0.803657 0.8098 0.816055 0.822424 0.828905 0.835498 0.842204 0.849023 0.855955 0.863 0.870157 0.877427 0.884809 0.892305 0.899913 0.907633 0.915467 0.923413 0.931472 0.939643 0.947927 0.956324 0.964834 0.973457 0.983281 0.983281 0.983281 0.983281
  arc A8 (2.2507, -1.3017) -> (2.2895, -1.2322) centre (0, 0) ccw